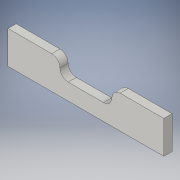
# Autodesk Inventor part: Drawer ends
Saved by Autodesk Inventor 2016 (Build 200138000, 138)
## iProperties
Created: 2017-10-31
Part Number: Drawer ends
Material: ABS Plastic
Document SubType Name: Modeling
Designer: mathaetaes
Density: 1.06 g/cm^3
Appearance: Smooth - White
Author: mathaetaes
Autodesk Inventor part; units mm, degrees
ref_plane "YZ Plane" through (0, 0, 0) normal (1, 0, 0) x (0, 1, 0)
ref_plane "XZ Plane" through (0, 0, 0) normal (0, 1, 0) x (-1, 0, 0)
ref_plane "XY Plane" through (0, 0, 0) normal (0, 0, 1) x (1, 0, 0)
sketch "Sketch1" plane through (0, 0, 0) normal (0, 0, 1) x (1, 0, 0)
  line L0 (-180.975, -30.3906) -> (180.975, -30.3906)
  line L1 (180.975, -30.3906) -> (180.975, -106.5906)
  line L2 (180.975, -106.5906) -> (-180.975, -106.5906)
  line L3 (-180.975, -106.5906) -> (-180.975, -30.3906)
  line L4 (0, 21.3181) -> (0, -127.9087) projected
  point P0 (0, 0)
  dimension "d0" = 361.95
  dimension "d1" = 76.2
  dimension "d4" = 180.975
  constraints: 8 end point, 2 parallel, 1 horizontal, 1 perpendicular
  measures "d0" distance of L1.end L2.end
  measures "d1" distance of L0.end L1.end
  measures "d4" distance between parallel lines of L1 L4
extrude "Extrusion1" add sketch "Sketch1" along normal blind 19.05
sketch "Sketch2" plane through (0, 0, 19.05) normal (0, 0, 1) x (1, 0, 0)
  line L0 (0, 21.3181) -> (0, -127.9087) projected
  line L1 (180.975, -30.3906) -> (-180.975, -30.3906) projected
  line L2 (-60.325, -30.3906) -> (60.325, -30.3906)
  line L3 (60.325, -30.3906) -> (60.325, -68.4906)
  line L4 (60.325, -68.4906) -> (-60.325, -68.4906)
  line L5 (-60.325, -68.4906) -> (-60.325, -30.3906)
  point P0 (0, 0)
  dimension "d5" = 120.65
  dimension "d6" = 60.325
  dimension "d7" = 38.1
  constraints: 8 end point, 2 parallel, 1 horizontal, 1 perpendicular, 1 point on line
  measures "d5" distance of L3.end L4.end
  measures "d6" distance between parallel lines of L5 L0
  measures "d7" distance of L2.end L3.end
extrude "Extrusion2" cut sketch "Sketch2" against normal blind 19.05
fillet "Fillet1" radius 19.05 4 edges at (-60.325, -30.3906, 9.525) (60.325, -30.3906, 9.525) (60.325, -68.4906, 9.525) (-60.325, -68.4906, 9.525)
equation "\"d4\" = 0.5 * d0"
equation "\"d5\" = 0.333333 * d0"
equation "\"d6\" = 0.5 * d5"
body "Solid1"
